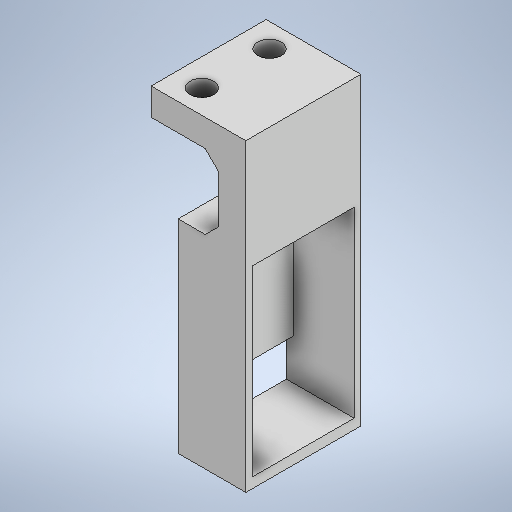
# Autodesk Inventor part: POUPLY_P6
Saved by Autodesk Inventor 2025 (Build 290162000, 162)
## iProperties
Created: 2024-04-13
Part Number: POUPLY_P6
Material: Générique
Document SubType Name: Modeling
Designer: chass
Density: 1 g/cm^3
Appearance: Par défaut
Author: chass
Autodesk Inventor part; units mm, degrees
ref_plane "YZ Plane" through (0, 0, 0) normal (1, 0, 0) x (0, 1, 0)
ref_plane "XZ Plane" through (0, 0, 0) normal (0, 1, 0) x (-1, 0, 0)
ref_plane "XY Plane" through (0, 0, 0) normal (0, 0, 1) x (1, 0, 0)
sketch "Esquisse1" plane through (0, 0, 0) normal (1, 0, 0) x (0, 1, 0)
  line L0 (15, 8.5) -> (-15, 8.5)
  line L1 (-15, 8.5) -> (-15, -8.5)
  line L2 (-15, -8.5) -> (15, -8.5)
  line L3 (15, -8.5) -> (15, 8.5)
  point P0 (0, 0)
  point P1 (0, 0)
  point P2 (0, 0)
  dimension "d4" = 30
  dimension "d5" = 17
  constraints: 8 end point, 2 parallel, 1 coincident, 1 horizontal, 1 perpendicular
  measures "d4" distance of L1.end L2.end
  measures "d5" distance of L2.end L0.start
extrude "Extrusion1" add sketch "Esquisse1" along normal blind 10
sketch "Esquisse2" plane through (10, 0, 0) normal (1, 0, 0) x (0, 0, -1)
  line L0 (-7.5, 13.5) -> (7.5, 13.5)
  line L1 (7.5, 13.5) -> (7.5, -13.5)
  line L2 (7.5, -13.5) -> (-7.5, -13.5)
  line L3 (-7.5, -13.5) -> (-7.5, 13.5)
  line L4 (-7.5, 13.5) -> (7.5, -13.5)
  line L5 (-7.5, -13.5) -> (7.5, 13.5)
  point P0 (0, 0)
  point P1 (0, 0)
  point P2 (0, 0)
  dimension "d8" = 27
  dimension "d9" = 15
  constraints: 12 end point, 2 midpoint, 2 parallel, 1 coincident, 1 horizontal, 1 perpendicular
  measures "d8" distance of L0.end L1.end
  measures "d9" distance of L0.start L0.end
extrude "Extrusion2" cut sketch "Esquisse2" against normal blind 9
sketch "Esquisse3" plane through (1, 0, 0) normal (1, 0, 0) x (0, 0, -1)
  line L0 (7.5, -13.5) -> (-7.5, -13.5) projected
  line L1 (7.5, 13.5) -> (7.5, -13.5) projected
  line L2 (-7.5, -13.5) -> (7.5, -13.5)
  line L3 (7.5, -13.5) -> (7.5, -7.5)
  line L4 (7.5, -7.5) -> (-7.5, -7.5)
  line L5 (-7.5, -7.5) -> (-7.5, -13.5)
  point P0 (0, 0)
  dimension "d12" = 6
  constraints: 8 end point, 2 parallel, 1 horizontal, 1 perpendicular, 1 point on line
  measures "d12" distance of L3.end L2.end
extrude "Extrusion3" cut sketch "Esquisse3" against normal blind 9
sketch "Esquisse9" plane through (0, 15, 8.5) normal (0, 1, 0) x (1, 0, 0)
  line L0 (0, 17) -> (10, 17) projected
  line L1 (0, 0) -> (10, 0) projected
  line L2 (10, 17) -> (6, 17)
  line L3 (6, 17) -> (6, 0)
  line L4 (6, 0) -> (10, 0)
  line L5 (10, 0) -> (10, 17)
  point P0 (0, 8.5)
  dimension "d58" = 4
  constraints: 8 end point, 2 parallel, 1 horizontal, 1 perpendicular, 1 point on line
  measures "d58" distance between parallel lines of L5 L3
extrude "Extrusion10" add sketch "Esquisse9" along normal blind 15
sketch "Esquisse10" plane through (6, 15, -8.5) normal (-1, 0, 0) x (0, 0, 1)
  line L0 (0, -30) -> (0, 15) projected
  line L1 (17, -30) -> (17, 15) projected
  line L2 (0, 15) -> (17, 15)
  line L3 (17, 15) -> (17, 11)
  line L4 (17, 11) -> (0, 11)
  line L5 (0, 11) -> (0, 15)
  point P0 (8.5, -15)
  point P1 (17, 15)
  point P2 (0, 11)
  dimension "d61" = 4
  constraints: 8 end point, 2 parallel, 1 horizontal, 1 perpendicular, 1 point on line
  measures "d61" distance between parallel lines of L2 L4
extrude "Extrusion11" add sketch "Esquisse10" along normal blind 10
chamfer "Chanfrein3" distance 2 angle 45 1 edges at (6, 26, 0)
chamfer "Chanfrein4" distance 2 angle 45 1 edges at (6, 15, 0)
sketch "Esquisse11" plane through (0, 30, 8.5) normal (0, 1, 0) x (1, 0, 0)
  line L0 (0, 17) -> (0, 0) projected
  circle A0 centre (0, 13.5) radius 1.75
  circle A1 centre (0, 3.5) radius 1.75
  line L1 (10, 17) -> (-4, 17) projected
  line L2 (0, 8.5) -> (10, 8.5) construction
  dimension "d70" = 3.5
  dimension "d71" = 3.5
  dimension "d72" = 10
  constraints: 2 centre point, 2 end point, 2 point on line, 1 horizontal, 1 symmetric about line
  measures "d70" diameter of A0
  measures "d71" diameter of A1
  measures "d72" distance of A0.centre A1.centre
extrude "Extrusion12" cut sketch "Esquisse11" against normal blind 10
